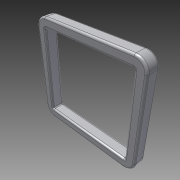
# Autodesk Inventor part: y_carryage_nut_holder_b_zip_tie
Saved by Autodesk Inventor 2014 (Build 180170000, 170)
## iProperties
Created: 2014-01-11
Part Number: y_carryage_nut_holder_b_zip_tie
Material: ABS Plastic
Document SubType Name: Modeling
Designer: buben
Density: 1.06 g/cm^3
Appearance: Smooth - White
Author: buben
Autodesk Inventor part; units mm, degrees
ref_plane "YZ Plane" through (0, 0, 0) normal (1, 0, 0) x (0, 1, 0)
ref_plane "XZ Plane" through (0, 0, 0) normal (0, 1, 0) x (-1, 0, 0)
ref_plane "XY Plane" through (0, 0, 0) normal (0, 0, 1) x (1, 0, 0)
sketch "Sketch1" plane through (0, 0, 0) normal (0, 1, 0) x (-1, 0, 0)
  line L0 (0.2, 0) -> (13.8, 0)
  line L1 (14, 0.2) -> (14, 12.8)
  line L2 (13.8, 13) -> (0.2, 13)
  line L3 (0, 12.8) -> (0, 0.2)
  arc A0 (0.2, 13) -> (0, 12.8) centre (0.2, 12.8) ccw
  arc A1 (14, 12.8) -> (13.8, 13) centre (13.8, 12.8) ccw
  arc A2 (13.8, 0) -> (14, 0.2) centre (13.8, 0.2) ccw
  arc A3 (0, 0.2) -> (0.2, 0) centre (0.2, 0.2) ccw
  line L4 (-1.5, 0.2) -> (-1.5, 12.8)
  arc A4 (0.2, 14.5) -> (-1.5, 12.8) centre (0.2, 12.8) ccw
  line L5 (0.2, 14.5) -> (13.8, 14.5)
  arc A5 (15.5, 12.8) -> (13.8, 14.5) centre (13.8, 12.8) ccw
  line L6 (15.5, 12.8) -> (15.5, 0.2)
  arc A6 (13.8, -1.5) -> (15.5, 0.2) centre (13.8, 0.2) ccw
  line L7 (13.8, -1.5) -> (0.2, -1.5)
  arc A7 (-1.5, 0.2) -> (0.2, -1.5) centre (0.2, 0.2) ccw
  point P0 (0, 0)
  dimension "d7" = 0.2
  dimension "d8" = 14
  dimension "d9" = 13
  dimension "d10" = 1.5
  constraints: 16 end point, 16 point on circle, 8 centre point, 8 tangent, 4 parallel, 3 equal radius, 2 perpendicular, 2 point on line, 1 horizontal, 7 other
  measures "d7" radius of A0
  measures "d8" distance between parallel lines of L1 L3
  measures "d9" distance between parallel lines of L0 L2
  measures "d10" distance between parallel lines of L4 L3
extrude "Extrusion1" add sketch "Sketch1" along normal blind 2
fillet "Fillet1" radius 0.3 32 edges at (1.0021, 2, 14.0021) (1.5, 2, 6.5) (1.0021, 2, -1.0021) (-7, 2, -1.5) (-15.0021, 2, -1.0021) (-15.5, 2, 6.5) (-15.0021, 2, 14.0021) (-7, 2, 14.5) (-13.9414, 2, 12.9414) (-14, 2, 6.5) (-13.9414, 2, 0.0586) (-7, 2, 0) (-0.0586, 2, 0.0586) (0, 2, 6.5) (-0.0586, 2, 12.9414) (-7, 2, 13) (-15.0021, 0, 14.0021) (-15.5, 0, 6.5) (-15.0021, 0, -1.0021) (-7, 0, -1.5) (1.0021, 0, -1.0021) (1.5, 0, 6.5) (1.0021, 0, 14.0021) (-7, 0, 14.5) (-0.0586, 0, 12.9414) (0, 0, 6.5) (-0.0586, 0, 0.0586) (-7, 0, 0) (-13.9414, 0, 0.0586) (-14, 0, 6.5) (-13.9414, 0, 12.9414) (-7, 0, 13)
body "Solid1"
